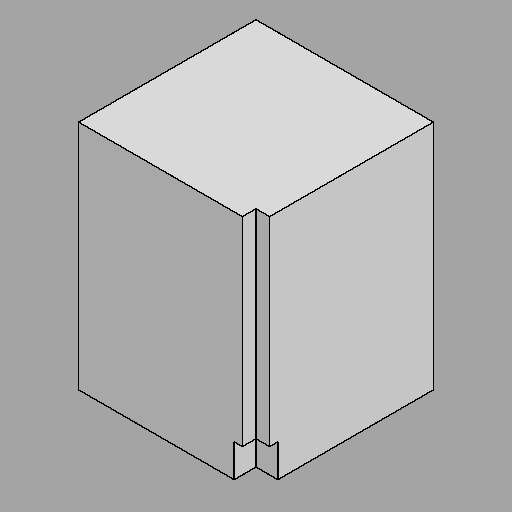
# Autodesk Inventor part: Mobile angolo
Saved by Autodesk Inventor 2025.2 (Build 292293000, 293)
## iProperties
Created: 2025-08-13
Part Number: Mobile angolo
Material: Generic
Document SubType Name: Modeling
Designer: Luca
Density: 1 g/cm^3
Appearance: Default
Mass: 356532 g
Surface Area: 30500 cm^2
Volume: 356532 cm^3
Mass: 635052 g
Surface Area: 46450 cm^2
Volume: 635052 cm^3
Author: Luca
FORNITO DA: ###
Autodesk Inventor part; units mm, degrees
ref_plane "YZ Plane" through (0, 0, 0) normal (1, 0, 0) x (0, 1, 0)
ref_plane "XZ Plane" through (0, 0, 0) normal (0, 1, 0) x (-1, 0, 0)
ref_plane "XY Plane" through (0, 0, 0) normal (0, 0, 1) x (1, 0, 0)
sketch "Sketch1" plane through (0, 0, 0) normal (0, 1, 0) x (1, 0, 0)
  line L0 (300, 0) -> (-300, 0)
  line L1 (-300, 0) -> (-300, -600)
  line L2 (-300, -600) -> (300, -600)
  line L3 (300, -600) -> (300, 0)
  point P0 (0, 0)
  point P1 (0, 0)
  dimension "d0" = 600
  dimension "d1" = 600
  constraints: 8 end point, 2 parallel, 1 coincident, 1 horizontal, 1 midpoint, 1 perpendicular
  measures "d0" distance of L1.end L2.end
  measures "d1" distance of L0.end L1.end
extrude "Extrusion1" add sketch "Sketch1" along normal blind 850
sketch "Sketch2" plane through (-300, 0, 600) normal (0, 0, 1) x (-1, 0, 0)
  line L0 (-600, 0) -> (-600, -850) projected
  line L1 (-600, 0) -> (-570, 0)
  line L2 (-570, 0) -> (-570, -120)
  line L3 (-570, -120) -> (-600, -120)
  line L4 (-600, -120) -> (-600, 0)
  point P0 (-300, 0)
  dimension "d4" = 120
  dimension "d7" = 30
  constraints: 8 end point, 2 parallel, 1 horizontal, 1 perpendicular
  measures "d4" distance of L2.end L1.end
  measures "d7" distance between parallel lines of L0 L2
extrude "Extrusion2" cut sketch "Sketch2" against normal blind 30
move faces "Move3" translate (50, 0, 0) faces at (300, 323.3333, 190)
move faces "Move4" translate (0, 0, 50) faces at (-110, 323.3333, 600)
sketch "Sketch3" plane through (270, 120, 570) normal (0, -1, 0) x (1, 0, 0)
  line L0 (-570, 80) -> (80, 80) projected
  line L1 (80, 80) -> (30, 80)
  line L2 (30, 80) -> (30, 30)
  line L3 (30, 30) -> (80, 30)
  line L4 (80, 30) -> (80, 80)
  line L5 (-570, 80) -> (-570, -570) projected
  line L6 (-570, -570) -> (80, -570) projected
  point P0 (-270, -570)
  dimension "d20" = 600
  dimension "d21" = 600
  constraints: 8 end point, 2 parallel, 1 horizontal, 1 perpendicular
  measures "d20" distance between parallel lines of L5 L2
  measures "d21" distance between parallel lines of L6 L3
extrude "Extrusion3" cut sketch "Sketch3" against normal through all
body "Solid1"
